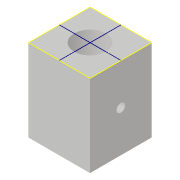
# Autodesk Inventor part: drill holder
Saved by Autodesk Inventor 2018 (Build 220112000, 112)
## iProperties
Created: 2019-01-18
Part Number: drill holder
Material: Generic
Document SubType Name: Modeling
Designer: ball
Density: 1 g/cm^3
Appearance: Default
Author: ball
Autodesk Inventor part; units mm, degrees
ref_plane "YZ Plane" through (0, 0, 0) normal (1, 0, 0) x (0, 1, 0)
ref_plane "XZ Plane" through (0, 0, 0) normal (0, 1, 0) x (-1, 0, 0)
ref_plane "XY Plane" through (0, 0, 0) normal (0, 0, 1) x (1, 0, 0)
sketch "Sketch1" plane through (0, 0, 0) normal (0, 1, 0) x (-1, 0, 0)
  line L0 (15.24, 9.525) -> (-3.81, 9.525)
  line L1 (-3.81, 9.525) -> (-3.81, -9.525)
  line L2 (-3.81, -9.525) -> (15.24, -9.525)
  line L3 (15.24, -9.525) -> (15.24, 9.525)
  point P0 (0, 0)
  dimension "d0" = 19.05
  dimension "d1" = 19.05
  constraints: 8 end point, 2 parallel, 1 horizontal, 1 perpendicular
  measures "d0" distance of L2.end L0.start
  measures "d1" distance of L1.end L2.end
extrude "Extrusion1" add sketch "Sketch1" along normal blind 25.4
sketch "Sketch2" plane through (0, 25.4, 0) normal (0, 1, 0) x (1, 0, 0)
  line L0 (-15.24, -9.525) -> (3.81, -9.525) projected
  line L1 (-5.715, -9.525) -> (-5.715, 9.525)
  line L2 (3.81, 9.525) -> (-15.24, 9.525) projected
  line L3 (-15.24, 9.525) -> (-15.24, -9.525) projected
  line L4 (-15.24, 0) -> (3.81, 0)
  line L5 (3.81, -9.525) -> (3.81, 9.525) projected
  point P0 (0, 0)
  constraints: 4 end point, 4 midpoint
sketch "Sketch3" plane through (0, 25.4, 0) normal (0, 1, 0) x (1, 0, 0)
  circle A0 centre (-5.715, 0) radius 4.8895 construction
  line L0 (3.81, -9.525) -> (3.81, 9.525) construction
  line L1 (3.81, 9.525) -> (-15.24, 9.525) construction
  circle A1 centre (-5.715, 0) radius 4.8895
  point P0 (0, 0)
  dimension "d4" = 9.779
  dimension "d5" = 9.525
  dimension "d6" = 9.525
  constraints: 2 centre point, 1 coincident, 1 concentric
  measures "d4" diameter of A0
  measures "d5" distance from line of L0 A0.centre
  measures "d6" distance from line of L1 A0.centre
extrude "Extrusion2" cut sketch "Sketch3" against normal through all
sketch "Sketch4" plane through (3.81, 0, 9.525) normal (1, 0, 0) x (0, 0, -1)
  circle A0 centre (9.525, 12.7) radius 1.3176
  line L0 (19.05, 0) -> (19.05, 25.4) projected
  line L1 (0, 25.4) -> (19.05, 25.4) projected
  point P0 (9.525, 0)
  dimension "d9" = 2.6353
  dimension "d10" = 9.525
  dimension "d11" = 12.7
  constraints: 1 centre point
  measures "d9" diameter of A0
  measures "d10" distance from line of L0 A0.centre
  measures "d11" distance from line of L1 A0.centre
extrude "Extrusion3" cut sketch "Sketch4" against normal through all
body "Solid1"
